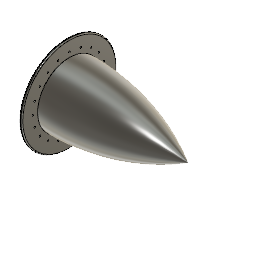
end_cone_eng_model (Autodesk Fusion 360 design; units mm, degrees)
Autodesk Fusion 360 part; units mm, degrees
sketch "Sketch1" plane through (0, 0, 0) normal (0, 1, 0) x (1, 0, 0)
  line L0 (284.8084, 0) -> (305, 0) construction
  line L1 (305, 0) -> (305, -120) construction
  line L2 (305, -120) -> (0, -120) construction
  line L3 (0, -120) -> (0, -69.9357) construction
  line L4 (0, -69.9357) -> (0, -120)
  line L5 (5, -120) -> (5, -80.02)
  line L6 (0, -120) -> (5, -120)
  arc A0 (5, -80.02) -> (305, 0) centre (11.9649, 496.2375) ccw
  arc A1 (0, -69.9357) -> (284.8084, 0) centre (11.9649, 496.2375) ccw
  line L7 (305, 0) -> (303.3901, 0)
  line L8 (305, 0) -> (300.6101, 0)
  line L9 (305, 0) -> (284.8084, 0)
  dimension "d1" = 120
  dimension "d3" = 5
  dimension "d5" = 80.02
  dimension "d6" = 305
  constraint horizontal L0
  constraint vertical L1
  constraint horizontal L2
  constraint vertical L3
  constraint coincident L2 L5.start
  constraint perpendicular L2 L5
  constraint concentric A0 A1
  constraint coincident L0 L7.end
  constraint coincident L0 L8.end
  measures "d1" distance of L0.end L1.end
  measures "d3" distance of L2.end L5.start
  measures "d5" vertical distance of origin L5.end
  measures "d6" distance of L1.end L2.end
revolve "Revolve1" add sketch "Sketch1" angle 360 about axis through (1.75, 0, 0) along (1, 0, 0)
fillet "Fillet1" radius 2.5 1 edges at (5, -43.3939, -111.8793)
sketch "Sketch2" plane through (0, 0, 0) normal (-1, 0, 0) x (0, -1, 0)
  circle A0 centre (0, 0) radius 120
  circle A1 centre (0, 0) radius 69.9357
  line L0 (0, 0) -> (0, 143.5123) construction
  circle A2 centre (0, 92) radius 2
  dimension "d11" = 4
  dimension "d12" = 92
  constraint coincident A0.centre A1.centre
  constraint vertical L0
  constraint coincident L0 A2.centre
  measures "d11" diameter of A2
  measures "d12" distance of A0.centre A2.centre
extrude "Extrude1" cut sketch "Sketch2" along normal mid plane 12 contours A2
pattern_circular "C-Pattern1" count 20 over 360 about axis through (1.75, 0, 0) along (1, 0, 0) of "Extrude1"
